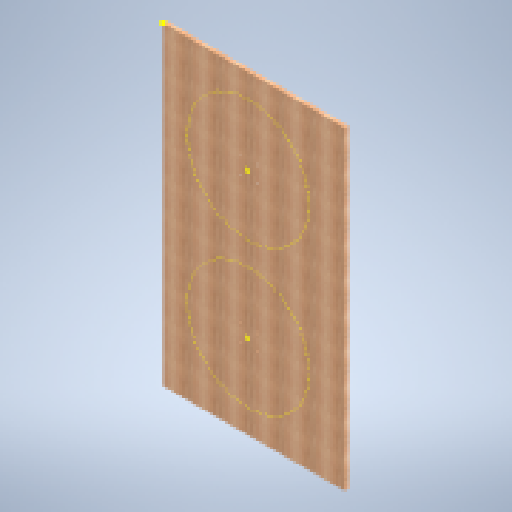
# Autodesk Inventor part: madeiraMesa
Saved by Autodesk Inventor 2023 (Build 270158000, 158)
## iProperties
Created: 2022-08-16
Part Number: madeiraMesa
Material: Generic
Document SubType Name: Modeling
Designer: cvss2
Density: 1 g/cm^3
Appearance: Default
largura: 2600,000 mm
comprimento: 1500,000 mm
Author: cvss2
Autodesk Inventor part; units mm, degrees
ref_plane "YZ Plane" through (0, 0, 0) normal (1, 0, 0) x (0, 1, 0)
ref_plane "XZ Plane" through (0, 0, 0) normal (0, 1, 0) x (-1, 0, 0)
ref_plane "XY Plane" through (0, 0, 0) normal (0, 0, 1) x (1, 0, 0)
sketch "Sketch1" plane through (0, 0, 0) normal (0, 0, 1) x (1, 0, 0)
  line L0 (0, 0) -> (1500, 0)
  line L1 (1500, 0) -> (1500, -2600)
  line L2 (1500, -2600) -> (0, -2600)
  line L3 (0, -2600) -> (0, 0)
  line L4 (682.5, -1882.5) -> (817.5, -1882.5) construction
  line L5 (817.5, -1882.5) -> (817.5, -2017.5) construction
  line L6 (817.5, -2017.5) -> (682.5, -2017.5) construction
  line L7 (682.5, -2017.5) -> (682.5, -1882.5) construction
  circle A0 centre (682.5, -1882.5) radius 5
  circle A1 centre (817.5, -1882.5) radius 5
  circle A2 centre (817.5, -2017.5) radius 5
  circle A3 centre (682.5, -2017.5) radius 5
  line L8 (682.5, -1882.5) -> (817.5, -2017.5) construction
  line L9 (817.5, -1882.5) -> (682.5, -2017.5) construction
  circle A4 centre (750, -1950) radius 505 construction
  circle A5 centre (750, -650) radius 505 construction
  line L10 (0, -1300) -> (1500, -1300) construction
  line L11 (682.5, -717.5) -> (817.5, -717.5) construction
  line L12 (817.5, -717.5) -> (817.5, -582.5) construction
  line L13 (817.5, -582.5) -> (682.5, -582.5) construction
  line L14 (682.5, -582.5) -> (682.5, -717.5) construction
  circle A6 centre (682.5, -717.5) radius 5
  circle A7 centre (817.5, -717.5) radius 5
  circle A8 centre (817.5, -582.5) radius 5
  circle A9 centre (682.5, -582.5) radius 5
  line L15 (682.5, -717.5) -> (817.5, -582.5) construction
  line L16 (817.5, -717.5) -> (682.5, -582.5) construction
  dimension "d0" = 1500
  dimension "d1" = 2600
  dimension "d4" = 135
  dimension "d5" = 135
  dimension "d6" = 10
  dimension "d7" = 10
  dimension "d8" = 10
  dimension "d9" = 10
  dimension "d10" = 1010
  dimension "d13" = 45
  dimension "d14" = 650
  dimension "d15" = 1010
  dimension "d16" = 650
  dimension "d17" = 750
  dimension "d18" = 750
  constraints: 34 end point, 10 centre point, 10 symmetric about line, 8 coincident, 4 parallel, 3 midpoint, 2 perpendicular, 2 point on line, 1 horizontal, 4 other
  measures "d0" distance of L1.end L2.end
  measures "d1" distance of L0.end L1.end
  measures "d4" distance of L5.end L6.end
  measures "d5" distance of L4.end L5.end
  measures "d6" diameter of A0
  measures "d7" diameter of A1
  measures "d8" diameter of A2
  measures "d9" diameter of A3
  measures "d10" diameter of A4
  measures "d13" angle of L6 L9
  measures "d14" distance from line of L2 A4.centre
  measures "d15" diameter of A5
  measures "d16" distance from line of L0 A5.centre
  measures "d17" distance from line of L1 A5.centre
  measures "d18" distance from line of L1 A4.centre
extrude "Extrusion1" add sketch "Sketch1" against normal blind 30
sketch "Sketch2" plane through (0, 0, 0) normal (0, 0, 1) x (1, 0, 0)
  circle A0 centre (750, -1950) radius 505 construction
  circle A1 centre (750, -650) radius 505 construction
  point P0 (0, 0)
equation "\"d0\" = comprimento"
equation "\"d1\" = largura"
equation "\"d7\" = d6"
equation "\"d8\" = d6"
equation "\"d9\" = d6"
equation "\"d14\" = distDenso"
equation "\"d15\" = d10"
equation "\"d16\" = d14"
equation "\"d17\" = d18"
equation "\"d18\" = 0.5 * d0"
equation "\"largura\" = 2600"
equation "\"comprimento\" = 1500"
equation "\"distDenso\" = 650"
body "Solid1"
